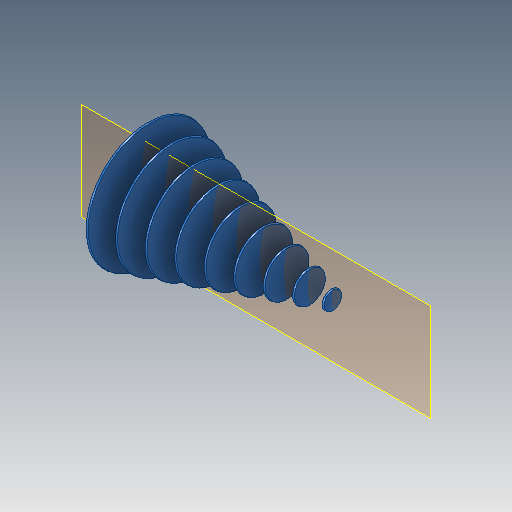
# Autodesk Inventor part: 00_light_inline_holography
Saved by Autodesk Inventor 2019.4 (Build 234330000, 330)
## iProperties
Created: 2019-11-29
Part Number: 00_light_inline_holography
Material: Glass
Document SubType Name: Modeling
Designer: marsikovabarbora
Density: 2.18 g/cm^3
Appearance: Cyan
Author: marsikovabarbora
Autodesk Inventor part; units mm, degrees
ref_plane "YZ Plane" through (0, 0, 0) normal (1, 0, 0) x (0, 1, 0)
ref_plane "XZ Plane" through (0, 0, 0) normal (0, 1, 0) x (-1, 0, 0)
ref_plane "XY Plane" through (0, 0, 0) normal (0, 0, 1) x (1, 0, 0)
ref_plane "Work Plane1" through (0, 0, 0) normal (0, 0, 1) x (1, 0, 0)
sketch "Sketch1" plane through (0, 0, 0) normal (0, 0, 1) x (1, 0, 0)
  line L0 (-140.04, 0) -> (-157.3007, 0) construction
  line L1 (-59.76, 0) -> (9.96, 0) construction
  line L2 (-32.3007, 16.8009) -> (-32.3007, -16.8009) construction
  line L3 (-32.3007, 16.8009) -> (-37.3007, 16.8009) construction
  line L4 (-37.3007, -16.8009) -> (-37.3007, 16.8009) construction
  line L5 (-32.3007, -16.8009) -> (-37.3007, -16.8009) construction
  line L6 (-180.5861, 13.4211) -> (-176.8, 13.4211) construction
  line L7 (-176.8, 13.635) -> (-176.8, 13.4211) construction
  line L8 (-175.4, 13.635) -> (-176.8, 13.635) construction
  line L9 (-175.4, 13.4211) -> (-175.4, 13.635) construction
  line L10 (-175.4, 13.4211) -> (-173.4, 13.4211) construction
  line L11 (-173.4, 16.635) -> (-173.4, 13.4211) construction
  line L12 (-188.8, 19.3504) -> (-173.4, 16.635) construction
  line L13 (-188.8, 9.135) -> (-188.8, 19.3504) construction
  line L14 (-188.8, 9.135) -> (-185.4, 9.135) construction
  line L15 (-185.4, 13.635) -> (-185.4, 9.135) construction
  line L16 (-180.8, 13.635) -> (-185.4, 13.635) construction
  line L17 (-180.5861, 13.4211) -> (-180.8, 13.635) construction
  line L18 (-179.9983, -3.665) -> (-179.9983, 3.935) construction
  line L19 (-32.3007, 0) -> (-51.5223, 5.5255)
  line L20 (-173.4, 0) -> (-172.3007, 0)
  arc A0 (-51.5223, 5.5255) -> (-52.3007, 0) centre (-32.3007, 0) ccw
  arc A1 (-52.4834, 5.8018) -> (-53.3007, 0) centre (-32.3007, 0) ccw
  arc A2 (-65.9385, 9.6697) -> (-67.3007, 0) centre (-32.3007, 0) ccw
  arc A3 (-66.8996, 9.946) -> (-68.3007, 0) centre (-32.3007, 0) ccw
  arc A4 (-80.3547, 13.8138) -> (-82.3007, 0) centre (-32.3007, 0) ccw
  arc A5 (-81.3157, 14.0901) -> (-83.3007, 0) centre (-32.3007, 0) ccw
  arc A6 (-94.7708, 17.958) -> (-97.3007, 0) centre (-32.3007, 0) ccw
  arc A7 (-95.7319, 18.2343) -> (-98.3007, 0) centre (-32.3007, 0) ccw
  arc A8 (-109.187, 22.1021) -> (-112.3007, 0) centre (-32.3007, 0) ccw
  arc A9 (-110.1481, 22.3784) -> (-113.3007, 0) centre (-32.3007, 0) ccw
  arc A10 (-123.6032, 26.2463) -> (-127.3007, 0) centre (-32.3007, 0) ccw
  arc A11 (-124.5642, 26.5226) -> (-128.3007, 0) centre (-32.3007, 0) ccw
  arc A12 (-138.0193, 30.3904) -> (-142.3007, 0) centre (-32.3007, 0) ccw
  arc A13 (-138.9804, 30.6667) -> (-143.3007, 0) centre (-32.3007, 0) ccw
  arc A14 (-152.4355, 34.5346) -> (-157.3007, 0) centre (-32.3007, 0) ccw
  arc A15 (-153.3966, 34.8109) -> (-158.3007, 0) centre (-32.3007, 0) ccw
  line L21 (-173.4, 0) -> (-173.4, 40.5612)
  arc A16 (-167.8128, 38.955) -> (-173.3007, 0) centre (-32.3007, 0) ccw
  arc A17 (-166.8517, 38.6787) -> (-172.3007, 0) centre (-32.3007, 0) ccw
  line L22 (-167.8128, 38.955) -> (-173.4, 40.5612)
  line L23 (-166.8517, 38.6787) -> (-167.8128, 38.955)
  line L24 (-153.3966, 34.8109) -> (-166.8517, 38.6787)
  line L25 (-152.4355, 34.5346) -> (-153.3966, 34.8109)
  line L26 (-138.9804, 30.6667) -> (-152.4355, 34.5346)
  line L27 (-138.0193, 30.3904) -> (-138.9804, 30.6667)
  line L28 (-124.5642, 26.5226) -> (-138.0193, 30.3904)
  line L29 (-123.6032, 26.2463) -> (-124.5642, 26.5226)
  line L30 (-110.1481, 22.3784) -> (-123.6032, 26.2463)
  line L31 (-109.187, 22.1021) -> (-110.1481, 22.3784)
  line L32 (-95.7319, 18.2343) -> (-109.187, 22.1021)
  line L33 (-94.7708, 17.958) -> (-95.7319, 18.2343)
  line L34 (-81.3157, 14.0901) -> (-94.7708, 17.958)
  line L35 (-66.8996, 9.946) -> (-80.3547, 13.8138)
  line L36 (-80.3547, 13.8138) -> (-81.3157, 14.0901)
  line L37 (-65.9385, 9.6697) -> (-66.8996, 9.946)
  line L38 (-52.4834, 5.8018) -> (-65.9385, 9.6697)
  line L39 (-51.5223, 5.5255) -> (-52.4834, 5.8018)
  line L40 (-172.3007, 0) -> (-158.3007, 0)
  line L41 (-158.3007, 0) -> (-143.3007, 0)
  line L42 (-157.3007, 0) -> (-209.76, 0) construction
  line L43 (-143.3007, 0) -> (-142.3007, 0)
  line L44 (-142.3007, 0) -> (-128.3007, 0)
  line L45 (-128.3007, 0) -> (-127.3007, 0)
  line L46 (-127.3007, 0) -> (-113.3007, 0)
  line L47 (-113.3007, 0) -> (-112.3007, 0)
  line L48 (-112.3007, 0) -> (-98.3007, 0)
  line L49 (-98.3007, 0) -> (-97.3007, 0)
  line L50 (-83.3007, 0) -> (-82.3007, 0)
  line L51 (-97.3007, 0) -> (-83.3007, 0)
  line L52 (-82.3007, 0) -> (-68.3007, 0)
  line L53 (-68.3007, 0) -> (-67.3007, 0)
  line L54 (-67.3007, 0) -> (-53.3007, 0)
  line L55 (-53.3007, 0) -> (-52.3007, 0)
  line L56 (-52.3007, 0) -> (-32.3007, 0)
  point P0 (0, 0)
  dimension "d0" = 1
  dimension "d1" = 1
  dimension "d2" = 1
  dimension "d3" = 1
  dimension "d4" = 1
  dimension "d5" = 1
  dimension "d6" = 1
  dimension "d7" = 1
  dimension "d9" = 20
  dimension "d10" = 35
  dimension "d11" = 50
  dimension "d12" = 65
  dimension "d13" = 80
  dimension "d14" = 95
  dimension "d15" = 110
  dimension "d16" = 125
  dimension "d17" = 1
  dimension "d18" = 140
  constraints: 62 end point, 36 point on circle, 18 centre point, 18 coincident, 16 point on line, 12 horizontal, 8 collinear, 1 midpoint, 1 vertical, 134 other
  measures "d0" radial gap between concentric circles of A1 A0
  measures "d1" radial gap between concentric circles of A2 A3
  measures "d2" radial gap between concentric circles of A4 A5
  measures "d3" radial gap between concentric circles of A6 A7
  measures "d4" radial gap between concentric circles of A8 A9
  measures "d5" radial gap between concentric circles of A10 A11
  measures "d6" radial gap between concentric circles of A12 A13
  measures "d7" radial gap between concentric circles of A14 A15
  measures "d9" radius of A0
  measures "d10" radius of A2
  measures "d11" radius of A4
  measures "d12" radius of A6
  measures "d13" radius of A8
  measures "d14" radius of A10
  measures "d15" radius of A12
  measures "d16" radius of A14
  measures "d17" radial gap between concentric circles of A17 A16
  measures "d18" radius of A17
revolve "Revolution1" add sketch "Sketch1" angle 360 about axis through (-82.3007, 0, 0) along (1, 0, 0) contours A0 L55 A1 L39 | A2 L53 A3 L37 | A4 L50 A5 L36 | A6 L49 A7 L33 | A8 L47 A9 L31 | A10 L45 A11 L29 | A12 L43 A13 L27 | A14 L41 A15 L25 | A17 L20 A16 L23
equation "\"d1\" = d0"
equation "\"d2\" = d0"
equation "\"d3\" = d0"
equation "\"d4\" = d0"
equation "\"d5\" = d0"
equation "\"d6\" = d0"
equation "\"d7\" = d0"
equation "\"d10\" = 1.75 * d9"
equation "\"d11\" = 2.5 * d9"
equation "\"d12\" = 3.25 * d9"
equation "\"d13\" = 4 * d9"
equation "\"d14\" = 4.75 * d9"
equation "\"d15\" = 5.5 * d9"
equation "\"d16\" = 6.25 * d9"
equation "\"d17\" = d0"
equation "\"d18\" = 7 * d9"
body "Solid1"
